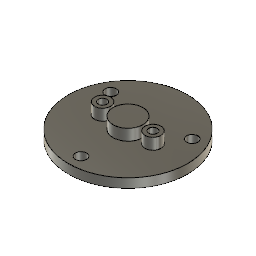
support_roulette_a_bille (Autodesk Fusion 360 design; units mm, degrees)
Autodesk Fusion 360 part; units mm, degrees
cylinder "CylinderPrimitive1" add diameter 32 height 2.5 placed x (1, 0, 0) y (0, 1, 0) z (0, 0, 1) at (0, 0, 0) makes body 1
sketch "Esquisse2" plane through (0, 0, 2.5) normal (0, 0, 1) x (-1, 0, 0)
  circle A0 centre (0, 0) radius 16
  circle A1 centre (0, 12.6) radius 1.5
  circle A2 centre (-10.9119, -6.3) radius 1.5
  circle A3 centre (10.9119, -6.3) radius 1.5
  dimension "d3" = 3
  dimension "d4" = 12.6
  dimension "d6" = 360
  measures "d3" diameter of A1
  measures "d4" distance of A0.centre A1.centre
extrude "Extrusion1" cut sketch "Esquisse2" against normal blind 3 contours A1 | A2 | A3 bodies 1
cylinder "CylinderPrimitive2" add diameter 8 height 3 placed x (1, 0, 0) y (0, 1, 0) z (0, 0, 1) at (0, 0, 2.5) bodies 1
cylinder "CylinderPrimitive3" add diameter 4.3 height 3 placed x (1, 0, 0) y (0, 1, 0) z (0, 0, 1) at (-7.2527, -0.0149, 2.5) separate body makes body 2
move_body "Déplacer1" bodies 2 to x (1, 0, 0) y (0, 1, 0) z (0, 0, 1) at (0.5067, -0.0419, 0)
mirror "Symétrie miroir1" about plane through (0, 0, 0) normal (1, 0, 0) of bodies 2 makes body 3
combine "Combiner1" operation add target body 2 tool bodies 3 1
hole "Perçage1" at (-6.746, -0.0568, 5.5) direction (0, 0, -1) diameter 2.3 depth 6 tip angle 118 bodies 2
hole "Perçage2" at (6.746, -0.0568, 5.5) direction (0, 0, -1) diameter 2.3 depth 6 tip angle 118 bodies 2
